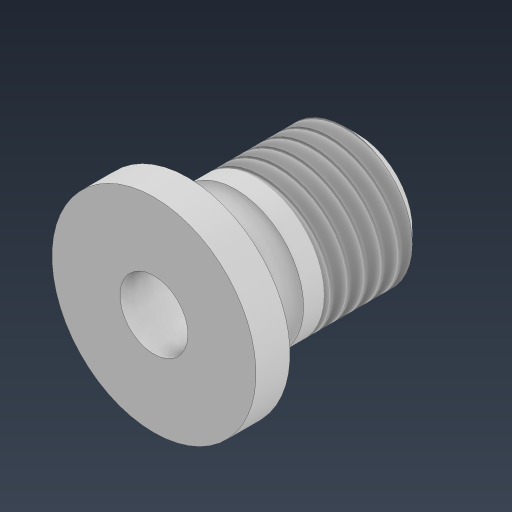
# Autodesk Inventor part: 3D Model
Saved by Autodesk Inventor 2024 (Build 280153000, 153)
## iProperties
Created: 2024-03-07
Part Number: 3D Model
Material: Genérico
Document SubType Name: Modeling
Designer: Administrator
Density: 1 g/cm^3
Appearance: Padrão
Author: Administrator
Autodesk Inventor part; units mm, degrees
ref_plane "YZ Plane" through (0, 0, 0) normal (1, 0, 0) x (0, 1, 0)
ref_plane "XZ Plane" through (0, 0, 0) normal (0, 1, 0) x (-1, 0, 0)
ref_plane "XY Plane" through (0, 0, 0) normal (0, 0, 1) x (1, 0, 0)
sketch "Esboço1" plane through (0, 0, 0) normal (1, 0, 0) x (0, 1, 0)
  line L0 (0, 0) -> (15, 0)
  line L1 (15, 0) -> (15, -5)
  line L2 (15, -5) -> (10, -5)
  line L3 (10, -30) -> (0, -30)
  line L4 (0, -30) -> (0, 0)
  line L5 (10, -5) -> (10, -8)
  arc A0 (10, -8) -> (10, -12) centre (10, -10) ccw
  line L6 (10, -12) -> (10, -30)
  point P0 (12.5, -5)
  point P1 (10, -6.5)
  dimension "d0" = 30
  dimension "d2" = 5
  dimension "d3" = 30
  dimension "d5" = 20
  dimension "d6" = 2
  dimension "d14" = 20
  constraints: 14 end point, 3 perpendicular, 2 midpoint, 2 point on circle, 2 point on line, 1 centre point, 1 collinear, 1 horizontal, 1 vertical
  measures "d0" diameter of L1 L4
  measures "d2" distance from line of point (12.5, -5) L0
  measures "d3" distance between parallel lines of L0 L3
  measures "d5" diameter of point (10, -6.5) L4
  measures "d6" radius of A0
  measures "d14" distance from line of L3 A0.centre
revolve "Revolução1" add sketch "Esboço1" angle 360 about axis through (0, 0, -30) along (0, 0, 1)
sketch "Esboço2" plane through (0, 0, -30) normal (0, 0, -1) x (-1, 0, 0)
  circle A0 centre (0, 0) radius 10 projected
  constraints: 1 coincident
hole "Furo1" at (0, 0, -30) direction (0, 0, 1) diameter 10 end through all
thread "Rosca1" size "M20x2.5" class "6g" standard "ANSI Metric M Profile" length 15
chamfer "Chanfro1" distance 2 angle 45 1 edges at (0, -10, -30)
